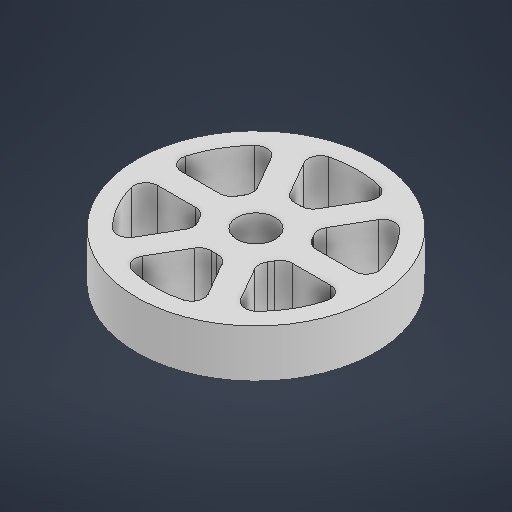
# Autodesk Inventor part: 2.5in flex
Saved by Autodesk Inventor 2025.2 (Build 292293000, 293)
## iProperties
Created: 2026-01-16
Part Number: 2.5in flex
Material: Generic
Document SubType Name: Modeling
Designer: cloudy
Density: 1 g/cm^3
Appearance: Default
Author: cloudy
Autodesk Inventor part; units mm, degrees
ref_plane "YZ Plane" through (0, 0, 0) normal (1, 0, 0) x (0, 1, 0)
ref_plane "XZ Plane" through (0, 0, 0) normal (0, 1, 0) x (-1, 0, 0)
ref_plane "XY Plane" through (0, 0, 0) normal (0, 0, 1) x (1, 0, 0)
sketch "Sketch1" plane through (0, 0, 0) normal (0, 1, 0) x (-1, 0, 0)
  circle A0 centre (0, 0) radius 31.75
  circle A1 centre (0, 0) radius 5.08
  line L0 (10.6493, 3.175) -> (26.8001, 3.175)
  line L1 (26.8001, -3.175) -> (10.6493, -3.175)
  line L2 (2.575, 10.81) -> (10.6504, 24.7971)
  line L3 (16.1497, 21.6221) -> (8.0743, 7.635)
  line L4 (-8.0743, 7.635) -> (-16.1497, 21.6221)
  line L5 (-10.6504, 24.7971) -> (-2.575, 10.81)
  line L6 (-10.6493, -3.175) -> (-26.8001, -3.175)
  line L7 (-26.8001, 3.175) -> (-10.6493, 3.175)
  line L8 (-2.575, -10.81) -> (-10.6504, -24.7971)
  line L9 (-16.1497, -21.6221) -> (-8.0743, -7.635)
  line L10 (8.0743, -7.635) -> (16.1497, -21.6221)
  line L11 (10.6504, -24.7971) -> (2.575, -10.81)
  arc A2 (10.6504, 24.7971) -> (-10.6504, 24.7971) centre (0, 0) ccw
  arc A3 (-16.1497, 21.6221) -> (-26.8001, 3.175) centre (0, 0) ccw
  arc A4 (-26.8001, -3.175) -> (-16.1497, -21.6221) centre (0, 0) ccw
  arc A5 (-10.6504, -24.7971) -> (10.6504, -24.7971) centre (0, 0) ccw
  arc A6 (16.1497, -21.6221) -> (16.1497, 21.6221) centre (0, 0) ccw
  arc A7 (10.6493, 3.175) -> (8.0743, 7.635) centre (0, 0) ccw
  arc A8 (2.575, 10.81) -> (-2.575, 10.81) centre (0, 0) ccw
  arc A9 (-8.0743, 7.635) -> (-10.6493, 3.175) centre (0, 0) ccw
  arc A10 (-10.6493, -3.175) -> (-8.0743, -7.635) centre (0, 0) ccw
  arc A11 (-2.575, -10.81) -> (2.575, -10.81) centre (0, 0) ccw
  arc A12 (8.0743, -7.635) -> (10.6493, -3.175) centre (0, 0) ccw
  dimension "d0" = 63.5
  dimension "d1" = 10.16
  dimension "d4" = 3.175
  dimension "d5" = 3.175
  dimension "d8" = 360
  dimension "d10" = 26.9875
  dimension "d11" = 11.1125
  constraints: 24 end point, 24 point on circle, 13 centre point, 4 coincident, 1 horizontal, 1 parallel, 37 other
  measures "d0" diameter of A0
  measures "d1" diameter of A1
  measures "d4" distance from line of point (0, 0) L0
  measures "d5" distance from line of point (0, 0) L1
  measures "d10" radius of A6
  measures "d11" radius of A12
extrude "Extrusion1" add sketch "Sketch1" along normal blind 12.7
fillet "Fillet1" radius 3.175 24 edges at (2.575, 6.35, 10.81) (-2.575, 6.35, 10.81) (-8.0743, 6.35, 7.635) (-10.6493, 6.35, 3.175) (-10.6493, 6.35, -3.175) (-8.0743, 6.35, -7.635) (-2.575, 6.35, -10.81) (2.575, 6.35, -10.81) (8.0743, 6.35, -7.635) (10.6493, 6.35, -3.175) (10.6493, 6.35, 3.175) (8.0743, 6.35, 7.635) (16.1497, 6.35, 21.6221) (10.6504, 6.35, 24.7971) (26.8001, 6.35, -3.175) (26.8001, 6.35, 3.175) (10.6504, 6.35, -24.7971) (16.1497, 6.35, -21.6221) (-16.1497, 6.35, -21.6221) (-10.6504, 6.35, -24.7971) (-26.8001, 6.35, -3.175) (-26.8001, 6.35, 3.175) (-16.1497, 6.35, 21.6221) (-10.6504, 6.35, 24.7971)
body "Solid1"
